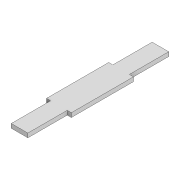
# Autodesk Inventor part: Gel wall
Saved by Autodesk Inventor 2020 (Build 240168000, 168)
## iProperties
Created: 2022-04-26
Part Number: Gel wall
Material: Generic
Document SubType Name: Modeling
Designer: ferrerx
Density: 1 g/cm^3
Appearance: Default
Author: ferrerx
Autodesk Inventor part; units mm, degrees
ref_plane "YZ Plane" through (0, 0, 0) normal (1, 0, 0) x (0, 1, 0)
ref_plane "XZ Plane" through (0, 0, 0) normal (0, 1, 0) x (-1, 0, 0)
ref_plane "XY Plane" through (0, 0, 0) normal (0, 0, 1) x (1, 0, 0)
sketch "Sketch1" plane through (0, 0, 0) normal (0, 1, 0) x (-1, 0, 0)
  line L0 (-10, 85) -> (10, 85)
  line L1 (10, 85) -> (10, -85)
  line L2 (10, -85) -> (-10, -85)
  line L3 (-10, -85) -> (-10, 85)
  line L4 (-10, 85) -> (10, -85) construction
  line L5 (10, 85) -> (-10, -85) construction
  point P0 (0, 0)
  dimension "d0" = 170
  dimension "d1" = 20
  constraints: 12 end point, 2 midpoint, 2 parallel, 1 horizontal, 1 perpendicular
  measures "d0" distance of L2.end L0.start
  measures "d1" distance of L1.end L2.end
extrude "Extrusion1" add sketch "Sketch1" along normal blind 5
sketch "Sketch2" plane through (0, 5, 0) normal (0, 1, 0) x (1, 0, 0)
  line L0 (0, 0) -> (10.5, 0)
  line L1 (6, -37.5) -> (15, -37.5)
  line L2 (15, -37.5) -> (15, 37.5)
  line L3 (15, 37.5) -> (6, 37.5)
  line L4 (6, 37.5) -> (6, -37.5)
  line L5 (6, -37.5) -> (15, 37.5) construction
  line L6 (15, -37.5) -> (6, 37.5) construction
  line L7 (10, -85) -> (10, 85) projected
  point P0 (10, 37.5)
  point P1 (10, -37.5)
  dimension "d4" = 5
  dimension "d5" = 75
  constraints: 14 end point, 2 horizontal, 2 midpoint, 2 parallel, 1 perpendicular, 1 other
  measures "d5" distance of L1.end L2.end
extrude "Extrusion2" add sketch "Sketch2" against normal blind 5 contours L7 L3 L2 L1
mirror "Mirror1" about plane through (0, 0, 0) normal (1, 0, 0) of "Extrusion2"
body "Solid1"
